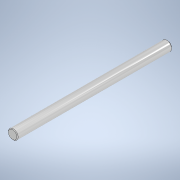
# Autodesk Inventor part: Fuehrungsschienen_Tension
Saved by Autodesk Inventor 2022 (Build 260153000, 153)
## iProperties
Created: 2023-07-31
Part Number: Fuehrungsschienen_Tension
Material: Aluminum 6061-AHC
Document SubType Name: Modeling
Designer: aewalder
Density: 2.7 g/cm^3
Appearance: Aluminum - Dark
Mass: 0.905573 g
Surface Area: 4.59502 cm^2
Volume: 0.335397 cm^3
Author: aewalder
Autodesk Inventor part; units mm, degrees
ref_plane "YZ Plane" through (0, 0, 0) normal (1, 0, 0) x (0, 1, 0)
ref_plane "XZ Plane" through (0, 0, 0) normal (0, 1, 0) x (-1, 0, 0)
ref_plane "XY Plane" through (0, 0, 0) normal (0, 0, 1) x (1, 0, 0)
sketch "Sketch1" plane through (0, 0, 0) normal (0, 0, 1) x (1, 0, 0)
  circle A0 centre (0, 0) radius 1.5
  dimension "d0" = 3
  constraints: 1 centre point, 1 coincident
  measures "d0" diameter of A0
extrude "Extrusion1" add sketch "Sketch1" along normal blind 47.5
chamfer "Chamfer1" distance 0.2 angle 45 2 edges at (-1.5, 0, 47.5) (-1.5, 0, 0)
body "Solid1"
